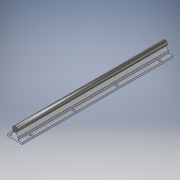
# Autodesk Inventor part: sbr12_350mm
Saved by Autodesk Inventor 2017 (Build 210142000, 142)
## iProperties
Created: 2016-06-20
Part Number: sbr12_350mm
Material: Generic
Document SubType Name: Modeling
Designer: brent
Density: 1 g/cm^3
Appearance: Aluminum - Flat
Author: brent
Autodesk Inventor part; units mm, degrees
ref_plane "YZ Plane" through (0, 0, 0) normal (1, 0, 0) x (0, 1, 0)
ref_plane "XZ Plane" through (0, 0, 0) normal (0, 1, 0) x (-1, 0, 0)
ref_plane "XY Plane" through (0, 0, 0) normal (0, 0, 1) x (1, 0, 0)
sketch "Sketch1" plane through (0, 0, 0) normal (0, 0, 1) x (1, 0, 0)
  circle A0 centre (0, 0) radius 6
  line L0 (-3, -5.1962) -> (-7.3323, -12.7)
  line L1 (-7.3323, -12.7) -> (7.3323, -12.7)
  line L2 (7.3323, -12.7) -> (3, -5.1962)
  line L3 (-7.5, -22.5) -> (7.5, -22.5)
  line L4 (7.5, -22.5) -> (7.5, -12.7)
  line L5 (7.5, -12.7) -> (-7.5, -12.7)
  line L6 (-7.5, -12.7) -> (-7.5, -22.5)
  line L7 (0, -12.7) -> (0, 0)
  line L8 (-17, -18) -> (17, -18)
  line L9 (17, -18) -> (17, -22.5)
  line L10 (17, -22.5) -> (-17, -22.5)
  line L11 (-17, -22.5) -> (-17, -18)
  point P0 (0, -22.5)
  dimension "d0" = 12
  dimension "d1" = 60
  dimension "d2" = 3
  dimension "d3" = 3
  dimension "d4" = 15
  dimension "d5" = 9.8
  dimension "d7" = 4.5
  dimension "d8" = 34
  dimension "d31" = 22.5
  constraints: 24 end point, 4 midpoint, 4 parallel, 3 horizontal, 2 perpendicular, 2 point on circle, 1 centre point, 1 coincident, 1 vertical
  measures "d0" diameter of A0
  measures "d1" angle of L2 L0
  measures "d2" horizontal distance of point (0, 0) L2.end
  measures "d3" horizontal distance of point (0, 0) L0.start
  measures "d4" distance of L5.end L4.end
  measures "d5" distance of L4.end L3.end
  measures "d7" distance of L8.end L9.end
  measures "d8" distance of L8.start L8.end
  measures "d31" distance from line of point (0, 0) L10
extrude "Extrusion1" add sketch "Sketch1" along normal blind 350
sketch "Sketch2" plane through (0, 0, 350) normal (0, 0, 1) x (1, 0, 0)
  arc A0 (3, -5.1962) -> (-3, -5.1962) centre (0, 0) ccw projected
  line L0 (3, -5.1962) -> (7.3323, -12.7) projected
  line L1 (7.3323, -12.7) -> (7.5, -12.7) projected
  line L2 (7.5, -12.7) -> (7.5, -18) projected
  line L3 (7.5, -18) -> (17, -18) projected
  line L4 (17, -18) -> (17, -22.5) projected
  line L5 (17, -22.5) -> (-17, -22.5) projected
  line L6 (-17, -22.5) -> (-17, -18) projected
  line L7 (-17, -18) -> (-7.5, -18) projected
  line L8 (-7.5, -18) -> (-7.5, -12.7) projected
  line L9 (-7.5, -12.7) -> (-7.3323, -12.7) projected
  line L10 (-7.3323, -12.7) -> (-3, -5.1962) projected
  line L11 (-6, -21.5) -> (6, -21.5)
  line L12 (6, -21.5) -> (6, -22.5)
  line L13 (6, -22.5) -> (-6, -22.5)
  line L14 (-6, -22.5) -> (-6, -21.5)
  point P0 (0, -22.5)
  dimension "d11" = 12
  dimension "d12" = 1
  constraints: 8 end point, 2 midpoint, 2 parallel, 1 horizontal, 1 perpendicular
  measures "d11" distance of L12.end L13.end
  measures "d12" distance of L11.end L12.end
extrude "Extrusion2" cut sketch "Sketch2" against normal through all contours L5 L14 L11 L12
chamfer "Chamfer1" distance 1 angle 45 2 edges at (-6, -21.5, 175) (6, -21.5, 175)
sketch "Sketch3" plane through (-17, -22.5, 0) normal (0, -1, 0) x (1, 0, 0)
  line L0 (23, 0) -> (23, 350) construction
  line L1 (23, 350) -> (34, 350) projected
  line L2 (34, 350) -> (34, 0) projected
  line L3 (34, 0) -> (23, 0) construction
  line L4 (11, 350) -> (11, 0) construction
  line L5 (11, 0) -> (0, 0) construction
  line L6 (0, 0) -> (0, 350) projected
  line L7 (0, 350) -> (11, 350) projected
  circle A0 centre (4.5, 25) radius 2.55
  circle A1 centre (29.5, 25) radius 2.55
  line L8 (29.5, 25) -> (4.5, 25) construction
  line L9 (17, 25) -> (17, 0) construction
  dimension "d18" = 25
  dimension "d19" = 5.1
  dimension "d20" = 5.1
  dimension "d21" = 25
  constraints: 4 end point, 2 centre point, 1 horizontal, 1 midpoint, 1 vertical
  measures "d18" distance of L9.start L9.end
  measures "d19" diameter of A1
  measures "d20" diameter of A0
  measures "d21" distance of L8.start L8.end
extrude "Extrusion3" cut sketch "Sketch3" against normal through all
pattern_linear "Rectangular Pattern1" count 4 spacing 100 along (0, 0, 1) of "Extrusion3"
sketch "Sketch4" plane through (0, 0, 0) normal (0, 0, -1) x (-1, 0, 0)
  line L0 (-5, -21.5) -> (-6, -22.5) projected
  line L1 (-5, -21.5) -> (5, -21.5) projected
  line L2 (6, -22.5) -> (5, -21.5) projected
  line L3 (17, -22.5) -> (6, -22.5) projected
  line L4 (17, -18) -> (17, -22.5) projected
  line L5 (7.5, -18) -> (17, -18) projected
  line L6 (7.5, -12.7) -> (7.5, -18) projected
  line L7 (7.3323, -12.7) -> (7.5, -12.7) projected
  line L8 (3, -5.1962) -> (7.3323, -12.7) projected
  arc A0 (3, -5.1962) -> (-3, -5.1962) centre (0, 0) ccw projected
  line L9 (-7.3323, -12.7) -> (-3, -5.1962) projected
  line L10 (-7.5, -12.7) -> (-7.3323, -12.7) projected
  line L11 (-7.5, -18) -> (-7.5, -12.7) projected
  line L12 (-17, -18) -> (-7.5, -18) projected
  line L13 (-17, -22.5) -> (-17, -18) projected
  line L14 (-6, -22.5) -> (-17, -22.5) projected
  circle A1 centre (0, 0) radius 6
  constraints: 1 coincident, 3 other
extrude "Extrusion4" cut sketch "Sketch4" against normal blind 0.5 contours A0 A1
sketch "Sketch5" plane through (0, 0, 350) normal (0, 0, 1) x (1, 0, 0)
  line L0 (6, -22.5) -> (17, -22.5) projected
  line L1 (17, -22.5) -> (17, -18) projected
  line L2 (17, -18) -> (7.5, -18) projected
  line L3 (7.5, -18) -> (7.5, -12.7) projected
  line L4 (7.5, -12.7) -> (7.3323, -12.7) projected
  line L5 (7.3323, -12.7) -> (3, -5.1962) projected
  arc A0 (3, -5.1962) -> (-3, -5.1962) centre (0, 0) ccw projected
  line L6 (-3, -5.1962) -> (-7.3323, -12.7) projected
  line L7 (-7.3323, -12.7) -> (-7.5, -12.7) projected
  line L8 (-7.5, -12.7) -> (-7.5, -18) projected
  line L9 (-7.5, -18) -> (-17, -18) projected
  line L10 (-17, -18) -> (-17, -22.5) projected
  line L11 (-17, -22.5) -> (-6, -22.5) projected
  line L12 (-5, -21.5) -> (-6, -22.5) projected
  line L13 (-5, -21.5) -> (5, -21.5) projected
  line L14 (6, -22.5) -> (5, -21.5) projected
  circle A1 centre (0, 0) radius 6
  constraints: 1 centre point, 1 coincident, 1 concentric
extrude "Extrusion5" cut sketch "Sketch5" against normal blind 0.5 contours A1 A0
body "Solid1"
